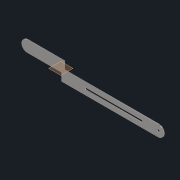
# Autodesk Inventor part: PalancaAccionMecBloq2
Saved by Autodesk Inventor 2021 (Build 250183000, 183)
## iProperties
Created: 2021-06-09
Part Number: PalancaAccionMecBloq2
Material: Stainless Steel
Document SubType Name: Modeling
Designer: GABRIEL LOL
Density: 8 g/cm^3
Appearance: Semi-Polished
Sheet Metal Width: 0.000 mm
Sheet Metal Length: 0.000 mm
Sheet Metal Area: 0.000 mm^2
Sheet Metal Rule: Default
Author: GABRIEL LOL
Autodesk Inventor part; units mm, degrees
ref_plane "YZ Plane" through (0, 0, 0) normal (1, 0, 0) x (0, 1, 0)
ref_plane "XZ Plane" through (0, 0, 0) normal (0, 1, 0) x (-1, 0, 0)
ref_plane "XY Plane" through (0, 0, 0) normal (0, 0, 1) x (1, 0, 0)
sketch "Sketch1" plane through (0, 0, 0) normal (0, 1, 0) x (-1, 0, 0)
  line L0 (0, 0) -> (184.2721, 0) construction
  line L1 (185, 0) -> (195.5441, 0) construction
  arc A0 (184.2721, 0) -> (184.2721, 0) centre (184.2721, -2) ccw
  arc A1 (192.5875, -13.3732) -> (192.5087, -14.1267) centre (194.5012, -13.9543) ccw
  line L2 (184.2721, 0) -> (0, 0)
  line L3 (184.2721, 0) -> (270, 0) construction
  line L4 (184.2721, 0) -> (194.5012, -13.9543)
  line L5 (194.5012, -13.9543) -> (270, -13.9543)
  point P0 (194.1925, -7.7135)
  dimension "d0" = 270
  dimension "d1" = 185
  dimension "d2" = 12
  dimension "d10" = 2
  constraints: 12 end point, 5 horizontal, 4 point on circle, 2 centre point, 2 point on line, 1 equal radius, 1 tangent
  measures "d0" distance of L0.start L3.end
  measures "d1" distance of L0.start L1.start
  measures "d2" distance of L1.start point (194.193, -7.713)
  measures "d10" radius of A0
sketch "Sketch2" plane through (0, 0, 0) normal (1, 0, 0) x (0, 1, 0)
  line L0 (0, 0) -> (20, 0)
  line L1 (20, 0) -> (20, -2)
  line L2 (20, -2) -> (0, -2)
  line L3 (0, -2) -> (0, 0)
  dimension "d4" = 20
  dimension "d5" = 2
  constraints: 8 end point, 2 parallel, 1 horizontal, 1 perpendicular
  measures "d4" distance of L1.end L2.end
  measures "d5" distance of L0.end L1.end
ref_plane "Work Plane1" through (-185, 20, 0) normal (0, 1, 0) x (1, 0, 0)
sweep "Sweep1" add profiles "Sketch2" path "Sketch1" path curves L2 L4 L5
sketch "Sketch5" plane through (-194.9205, 0, -2) normal (0, 0, -1) x (-1, 0, 0)
  line L0 (0, 20) -> (0, 0) projected
  line L1 (0, 0) -> (97.0795, 0) projected
  line L2 (97.0795, 20) -> (97.0795, 0) projected
  line L3 (0, 20) -> (97.0795, 20) projected
  line L4 (-194.9205, 0) -> (-194.9205, 20) projected
  line L5 (-194.9205, 0) -> (-11.6621, 0) projected
  line L6 (-194.9205, 20) -> (-11.6621, 20) projected
  circle A0 centre (87.0795, 10) radius 10
  circle A1 centre (-184.9205, 10) radius 10
  line L7 (-11.6621, 20) -> (-11.6621, 0) projected
  point P0 (-194.9205, 10)
  point P1 (-184.9205, 20)
  point P2 (-184.9205, 0)
  constraints: 6 tangent, 2 centre point
extrude "Extrusion2" cut sketch "Sketch5" against normal blind 10 contours L4 A1 L5 | L4 L6 A1
sketch "Sketch6" plane through (-183.2583, 0, -2) normal (0, 0, -1) x (-1, 0, 0)
  arc A0 (-173.2583, 20) -> (-173.2583, 0) centre (-173.2583, 10) ccw construction
  line L0 (-183.2583, 10) -> (-143.2583, 10) construction
  line L1 (-143.2583, 10) -> (-43.2583, 10) construction
  line L2 (-43.2583, 10) -> (-143.2583, 10) construction
  line L3 (-43.2583, 12) -> (-143.2583, 12)
  line L4 (-143.2583, 8) -> (-43.2583, 8)
  arc A1 (-43.2583, 8) -> (-43.2583, 12) centre (-43.2583, 10) ccw
  arc A2 (-143.2583, 12) -> (-143.2583, 8) centre (-143.2583, 10) ccw
  point P0 (-183.2583, 0)
  point P1 (-93.2583, 10)
  dimension "d15" = 40
  dimension "d16" = 100
  dimension "d17" = 4
  constraints: 12 end point, 5 point on circle, 4 tangent, 2 centre point, 2 horizontal, 1 collinear, 1 midpoint, 1 parallel
  measures "d15" distance of L0.start L0.end
  measures "d16" distance of L0.end L1.end
  measures "d17" diameter of A2
extrude "Extrusion3" cut sketch "Sketch6" against normal blind 10
sketch "Sketch7" plane through (-183.2583, 0, -2) normal (0, 0, -1) x (-1, 0, 0)
  arc A0 (-173.2583, 20) -> (-173.2583, 0) centre (-173.2583, 10) ccw construction
  line L0 (-183.2583, 10) -> (-173.2583, 10) construction
  circle A1 centre (-173.2583, 10) radius 2.5
  point P0 (-183.2583, 0)
  dimension "d20" = 5
  constraints: 2 end point, 1 centre point, 1 coincident, 1 horizontal, 1 point on circle
  measures "d20" diameter of A1
extrude "Extrusion4" cut sketch "Sketch7" against normal blind 10
sketch "Sketch8" plane through (-270, 0, -2) normal (0, 0, -1) x (-1, 0, 0)
  circle A0 centre (-260, 10) radius 2.5 projected
  line L0 (-130, 8) -> (-230, 8) projected
  arc A1 (-230, 12) -> (-230, 8) centre (-230, 10) ccw projected
  line L1 (-230, 12) -> (-130, 12) projected
  arc A2 (-130, 8) -> (-130, 12) centre (-130, 10) ccw projected
  arc A3 (-260, 20) -> (-260, 0) centre (-260, 10) ccw projected
  line L2 (-260, 0) -> (-86.7417, 0) projected
  line L3 (-260, 20) -> (-86.7417, 20) projected
  line L4 (-260, 20) -> (-85.7279, 20) projected
  line L5 (-120.2298, 20) -> (-120.2298, 0)
  line L6 (-260, 0) -> (-85.7279, 0) projected
  line L7 (-86.7417, 20) -> (-86.7417, 0) projected
  point P0 (-270, 0)
  point P1 (0, 0)
  point P2 (0, 20)
  constraints: 2 end point, 2 point on line, 1 perpendicular
sketch "Sketch9" plane through (-270, 20, -13.9543) normal (0, 0, 1) x (1, 0, 0)
  line L0 (0, 0) -> (0, -20) construction
  line L1 (0, -10) -> (10, -10) construction
  line L2 (75.4988, 0) -> (0, 0) projected
  arc A0 (10, 0) -> (10, -20) centre (10, -10) ccw
  line L3 (76.5125, -20) -> (0, -20) projected
  line L4 (10, -20) -> (0, -20)
  line L5 (0, -20) -> (0, 0)
  line L6 (0, 0) -> (10, 0)
  point P0 (270, -20)
  dimension "d23" = 10
  constraints: 8 end point, 3 point on circle, 2 horizontal, 1 centre point, 1 collinear, 1 midpoint, 1 point on line
  measures "d23" distance of L1.start L1.end
extrude "Extrusion5" cut sketch "Sketch9" against normal blind 10
equation "\"BendRadius\" = Thickness"
equation "\"BendReliefWidth\" = Thickness"
equation "\"BendReliefDepth\" = 0.5 * Thickness"
equation "\"CornerReliefSize\" = 4 * Thickness"
equation "\"MinimumRemnant\" = 2 * Thickness"
equation "\"TransitionRadius\" = BendRadius"
equation "\"JacobiRadiusSize\" = Thickness"
equation "\"GapSize\" = Thickness"
equation "\"Thickness\" = 0.5"
body "Solid2"
